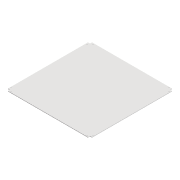
# Autodesk Inventor part: 底板
Saved by Autodesk Inventor 2021 (Build 250183000, 183)
## iProperties
Created: 2025-04-16
Part Number: 底板
Material: 常规
Document SubType Name: Modeling
Designer: 86155
Density: 1 g/cm^3
Appearance: 默认
Author: 86155
Autodesk Inventor part; units mm, degrees
ref_plane "YZ Plane" through (0, 0, 0) normal (1, 0, 0) x (0, 1, 0)
ref_plane "XZ Plane" through (0, 0, 0) normal (0, 1, 0) x (-1, 0, 0)
ref_plane "XY Plane" through (0, 0, 0) normal (0, 0, 1) x (1, 0, 0)
sketch "草图1" plane through (0, 0, 0) normal (0, 1, 0) x (-1, 0, 0)
  line L0 (0, 0) -> (-820, 0)
  line L1 (-820, 0) -> (-820, -820)
  line L2 (-820, -820) -> (0, -820)
  line L3 (0, -820) -> (0, 0)
  dimension "d0" = 820
  dimension "d1" = 820
  constraints: 8 end point, 2 parallel, 1 horizontal, 1 perpendicular
  measures "d0" distance of L2.end L1.end
  measures "d1" distance of L1.end L0.end
extrude "拉伸1" add sketch "草图1" along normal blind 5
sketch "草图2" plane through (0, 5, 0) normal (0, 1, 0) x (1, 0, 0)
  line L0 (0, 0) -> (820, 0) projected
  line L1 (0, 0) -> (20, 0)
  line L2 (20, 0) -> (20, 20)
  line L3 (20, 20) -> (0, 20)
  line L4 (0, 20) -> (0, 0)
  line L5 (820, 0) -> (800, 0)
  line L6 (800, 0) -> (800, 20)
  line L7 (800, 20) -> (820, 20)
  line L8 (820, 20) -> (820, 0)
  line L9 (820, 820) -> (0, 820) projected
  line L10 (820, 820) -> (800, 820)
  line L11 (800, 820) -> (800, 800)
  line L12 (800, 800) -> (820, 800)
  line L13 (820, 800) -> (820, 820)
  line L14 (0, 820) -> (20, 820)
  line L15 (20, 820) -> (20, 800)
  line L16 (20, 800) -> (0, 800)
  line L17 (0, 800) -> (0, 820)
  dimension "d4" = 20
  dimension "d5" = 20
  dimension "d6" = 20
  dimension "d7" = 20
  dimension "d8" = 20
  dimension "d9" = 20
  dimension "d10" = 20
  dimension "d11" = 20
  constraints: 32 end point, 8 parallel, 4 horizontal, 4 perpendicular
  measures "d4" distance of L3.end L2.end
  measures "d5" distance of L2.end L1.end
  measures "d6" distance of L6.end L7.end
  measures "d7" distance of L5.end L6.end
  measures "d8" distance of L12.end L11.end
  measures "d9" distance of L11.end L10.end
  measures "d10" distance of L15.end L16.end
  measures "d11" distance of L14.end L15.end
extrude "拉伸2" cut sketch "草图2" against normal blind 5
sketch "草图3" plane through (0, 5, 0) normal (0, 1, 0) x (1, 0, 0)
  line L0 (20, 0) -> (800, 0) projected
  line L1 (0, 800) -> (0, 20) projected
  line L2 (820, 20) -> (820, 800) projected
  line L3 (800, 820) -> (20, 820) projected
  point P0 (0, 0)
  point P1 (40, 10)
  point P2 (780, 10)
  point P3 (810, 780)
  point P4 (780, 810)
  point P5 (40, 810)
  point P6 (10, 780)
  point P7 (10, 40)
  point P8 (810, 40)
  dimension "d14" = 10
  dimension "d15" = 40
  dimension "d16" = 10
  dimension "d17" = 40
  dimension "d18" = 10
  dimension "d19" = 40
  dimension "d20" = 10
  dimension "d21" = 40
  dimension "d22" = 10
  dimension "d23" = 40
  dimension "d24" = 10
  dimension "d25" = 40
  dimension "d26" = 10
  dimension "d27" = 40
  dimension "d28" = 10
  dimension "d29" = 40
  measures "d14" distance from line of L0 point (40, 10)
  measures "d15" distance from line of L1 point (40, 10)
  measures "d16" distance from line of L0 point (780, 10)
  measures "d17" distance from line of L2 point (780, 10)
  measures "d18" distance from line of L2 point (810, 40)
  measures "d19" distance from line of L0 point (810, 40)
  measures "d20" distance from line of L2 point (810, 780)
  measures "d21" distance from line of L3 point (810, 780)
  measures "d22" distance from line of L3 point (780, 810)
  measures "d23" distance from line of L2 point (780, 810)
  measures "d24" distance from line of L3 point (40, 810)
  measures "d25" distance from line of L1 point (40, 810)
  measures "d26" distance from line of L1 point (10, 780)
  measures "d27" distance from line of L3 point (10, 780)
  measures "d28" distance from line of L1 point (10, 40)
  measures "d29" distance from line of L0 point (10, 40)
hole "孔1" at (40, 5, -10) at (780, 5, -10) at (810, 5, -780) at (780, 5, -810) at (40, 5, -810) at (10, 5, -780) at (10, 5, -40) at (810, 5, -40) direction (0, -1, 0) diameter 4.9587 depth 13.8 tip angle 118 thread size "M5.5x0.5" class "6H" standard "GB Metric profile"
sketch "草图5" plane through (0, 5, 0) normal (0, 1, 0) x (1, 0, 0)
  circle A0 centre (410, 410) radius 300
  line L0 (820, 20) -> (820, 800) projected
  line L1 (800, 820) -> (20, 820) projected
  line L2 (410, 410) -> (710, 410)
  circle A1 centre (410, 410) radius 300
  circle A2 centre (410, 410) radius 300
  circle A3 centre (410, 410) radius 300
  point P0 (0, 0)
  point P1 (410, 710)
  point P2 (410, 710)
  point P3 (110, 410)
  point P4 (110, 410)
  point P5 (410, 110)
  point P6 (410, 110)
  dimension "d57" = 600
  dimension "d58" = 410
  dimension "d59" = 410
  dimension "d62" = 360
  constraints: 6 coincident, 2 end point, 2 horizontal alignment, 2 vertical alignment, 1 horizontal, 23 other
  measures "d58" distance from line of L0 L2.start
  measures "d59" distance from line of L1 L2.start
hole "孔3" at (710, 5, -410) at (410, 5, -710) at (110, 5, -410) at (410, 5, -110) direction (0, -1, 0) diameter 9.188 depth 24 tip angle 118 thread size "M10x0.75" class "6H" standard "GB Metric profile"
